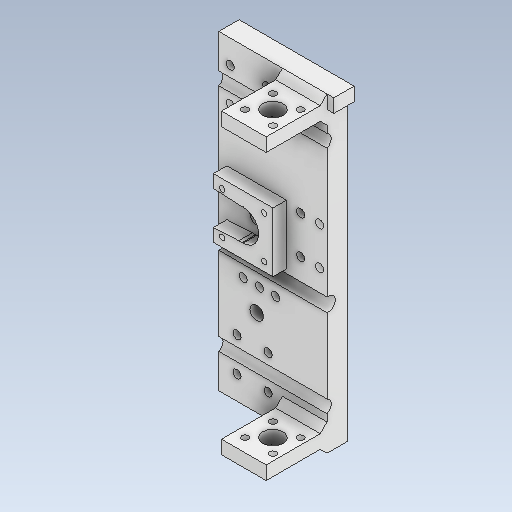
# Autodesk Inventor part: 0008-10-009 X Axis suport
Saved by Autodesk Inventor 2020 (Build 240168000, 168)
## iProperties
Created: 2021-02-27
Part Number: 0008-10-009 X Axis suport
Material: ABS Plastic
Document SubType Name: Modeling
Designer: Iulian Bors
Density: 1.06 g/cm^3
Appearance: Smooth - White
Mass: 294.815 g
Surface Area: 644.248 cm^2
Volume: 278.127 cm^3
Description: Supăort Axa X
Author: Iulian Bors
Subject: 009
Autodesk Inventor part; units mm, degrees
ref_plane "YZ Plane" through (0, 0, 0) normal (1, 0, 0) x (0, 1, 0)
ref_plane "XZ Plane" through (0, 0, 0) normal (0, 1, 0) x (-1, 0, 0)
ref_plane "XY Plane" through (0, 0, 0) normal (0, 0, 1) x (1, 0, 0)
sketch "Sketch1" plane through (0, 0, 0) normal (0, 0, 1) x (1, 0, 0)
  line L0 (-40, 115) -> (40, 115)
  line L1 (40, 115) -> (40, -115)
  line L2 (40, -115) -> (-40, -115)
  line L3 (-40, -115) -> (-40, 115)
  point P0 (0, 0)
  point P1 (0, 115)
  point P2 (-40, 0)
  dimension "d0" = 230
  dimension "d1" = 80
  constraints: 8 end point, 2 midpoint, 2 parallel, 1 horizontal, 1 horizontal alignment, 1 perpendicular, 1 vertical alignment
  measures "d0" distance of L2.end L0.start
  measures "d1" distance of L1.end L2.end
extrude "Extrusion1" add sketch "Sketch1" along normal blind 15
sketch "Sketch2" plane through (40, -115, 0) normal (1, 0, 0) x (0, 0, -1)
  circle A0 centre (-17, 30) radius 5.15
  circle A1 centre (-17, 200) radius 5.15
  line L0 (-15, 0) -> (-15, 230) projected
  line L1 (0, 230) -> (-15, 230) projected
  line L2 (0, 0) -> (-15, 0) projected
  point P0 (0, 115)
  dimension "d4" = 10.3
  dimension "d5" = 2
  dimension "d6" = 30
  dimension "d7" = 2
  dimension "d8" = 30
  constraints: 2 centre point, 1 equal radius
  measures "d4" diameter of A1
  measures "d5" distance from line of L0 A1.centre
  measures "d6" distance from line of L1 A1.centre
  measures "d7" distance from line of A0.centre L0
  measures "d8" distance from line of A0.centre L2
extrude "Extrusion2" cut sketch "Sketch2" against normal through all
sketch "Sketch3" plane through (-40, -115, 0) normal (-1, 0, 0) x (0, 0, 1)
  circle A0 centre (14, 95) radius 5.15
  line L0 (15, 195.2542) -> (15, 34.7458) projected
  line L1 (0, 0) -> (15, 0) projected
  point P0 (0, 115)
  dimension "d11" = 1
  dimension "d12" = 10.3
  dimension "d13" = 95
  constraints: 1 centre point
  measures "d11" distance from line of L0 A0.centre
  measures "d12" diameter of A0
  measures "d13" distance from line of A0.centre L1
extrude "Extrusion3" cut sketch "Sketch3" against normal through all
sketch "Sketch5" plane through (0, 0, 0) normal (0, 0, -1) x (-1, 0, 0)
  line L0 (34, -12) -> (-10, -12)
  line L1 (-10, -12) -> (-10, 32)
  line L2 (-10, 32) -> (34, 32)
  line L3 (34, 32) -> (34, -12)
  line L4 (34, -12) -> (-10, 32) construction
  line L5 (-10, -12) -> (34, 32) construction
  line L6 (-40, -115) -> (-40, 115)
  line L7 (-40, 115) -> (40, 115) projected
  line L8 (40, -115) -> (-40, -115) projected
  line L9 (-40, -115) -> (-40, 115) projected
  point P0 (12, 10)
  point P1 (12, -12)
  point P2 (0, -115)
  dimension "d17" = 44
  dimension "d43" = 105
  dimension "d64" = 52
  constraints: 14 end point, 4 midpoint, 3 perpendicular, 2 parallel
  measures "d17" distance of L0.start L0.end
  measures "d43" distance from line of L7 point (12, 10)
  measures "d64" distance from line of L6 point (12, 10)
extrude "Extrusion4" cut sketch "Sketch5" against normal blind 10
sketch "Sketch6" plane through (0, 0, 10) normal (0, 0, -1) x (-1, 0, 0)
  circle A0 centre (12, 10) radius 12.5
  line L0 (-40, -115) -> (-40, 115) projected
  line L1 (-40, 115) -> (40, 115) projected
  line L2 (40, -115) -> (-40, -115) projected
  point P0 (0, -115)
  dimension "d20" = 25
  dimension "d45" = 105
  dimension "d65" = 52
  constraints: 1 centre point, 1 coincident, 1 midpoint
  measures "d20" diameter of A0
  measures "d45" distance from line of L1 point (12, 10)
  measures "d65" distance from line of L0 point (12, 10)
extrude "Extrusion5" cut sketch "Sketch6" against normal blind 3
sketch "Sketch7" plane through (-12, 10, 13) normal (0, 0, -1) x (-1, 0, 0)
  circle A0 centre (0, 0) radius 5
  line L0 (-52, -125) -> (-52, 105) projected
  line L1 (-52, 105) -> (28, 105) projected
  line L2 (28, -125) -> (-52, -125) projected
  point P0 (-12, -125)
  dimension "d23" = 10
  dimension "d49" = 105
  dimension "d66" = 52
  constraints: 1 centre point, 1 coincident, 1 midpoint
  measures "d23" diameter of A0
  measures "d49" distance from line of L1 point (0, 0)
  measures "d66" distance from line of L0 point (0, 0)
extrude "Extrusion6" cut sketch "Sketch7" against normal through all
sketch "Sketch8" plane through (0, 0, 15) normal (0, 0, 1) x (1, 0, 0)
  line L0 (3.5, 25.5) -> (-27.5, 25.5) construction
  line L1 (-27.5, 25.5) -> (-27.5, -5.5) construction
  line L2 (-27.5, -5.5) -> (3.5, -5.5) construction
  line L3 (3.5, -5.5) -> (3.5, 25.5) construction
  line L4 (3.5, 25.5) -> (-27.5, -5.5) construction
  line L5 (-27.5, 25.5) -> (3.5, -5.5) construction
  line L6 (40, -115) -> (40, 115) projected
  line L7 (40, 115) -> (-40, 115) projected
  line L8 (-40, -115) -> (40, -115) projected
  point P0 (-12, 10)
  point P1 (-12, 10)
  point P2 (0, -115)
  dimension "d26" = 31
  dimension "d47" = 105
  dimension "d67" = 52
  constraints: 12 end point, 5 coincident, 3 midpoint, 2 parallel, 2 perpendicular, 1 horizontal
  measures "d26" distance of L1.end L2.end
  measures "d47" distance from line of L7 point (-12, 10)
  measures "d67" distance from line of point (-12, 10) L6
hole "Hole1" at (3.5, -5.5, 15) at (-27.5, -5.5, 15) at (-27.5, 25.5, 15) at (3.5, 25.5, 15) direction (0, 0, -1) diameter 4 depth 8 tip angle 118
sketch "Sketch9" plane through (0, 0, 15) normal (0, 0, 1) x (1, 0, 0)
  circle A0 centre (-27.5, 25.5) radius 2 projected
  circle A1 centre (3.5, -5.5) radius 2 projected
  circle A2 centre (-27.5, -5.5) radius 2
  circle A3 centre (3.5, 25.5) radius 2 projected
  circle A4 centre (-12, 10) radius 5
  line L0 (40, -25.052) -> (-40, -25.052) projected
  line L1 (-40, -25.052) -> (-40, -80.2542) projected
  line L2 (-40, -80.2542) -> (40, -80.2542) projected
  line L3 (40, -80.2542) -> (40, -25.052) projected
  line L4 (40, 80.2542) -> (-40, 80.2542) projected
  line L5 (-40, 80.2542) -> (-40, -14.948) projected
  line L6 (-40, -14.948) -> (40, -14.948) projected
  line L7 (40, 115) -> (-40, 115) projected
  line L8 (10, -12) -> (-34, -12)
  line L9 (-34, -12) -> (-34, 32)
  line L10 (-34, 32) -> (10, 32)
  line L11 (10, 32) -> (10, -12)
  line L12 (10, -12) -> (-34, 32) construction
  line L13 (-34, -12) -> (10, 32) construction
  line L14 (40, -14.948) -> (40, 80.2542) projected
  line L15 (-40, -115) -> (40, -115)
  line L16 (-40, -14.948) -> (40, -14.948) projected
  point P0 (-12, 10)
  point P1 (-12, -12)
  point P2 (0, -115)
  point P3 (10, 10)
  dimension "d52" = 105
  dimension "d55" = 44
  dimension "d68" = 52
  dimension "d69" = 44
  constraints: 14 end point, 6 midpoint, 3 perpendicular, 2 centre point, 2 parallel, 1 coincident, 1 horizontal, 1 horizontal alignment
  measures "d52" distance from line of L7 A4.centre
  measures "d55" distance of L8.start L8.end
  measures "d68" distance from line of A4.centre L14
  measures "d69" distance of L10.end L8.start
extrude "Extrusion7" add sketch "Sketch9" along normal blind 10 contours L8 L9 L10 L11
sketch "Sketch10" plane through (0, 0, 25) normal (0, 0, 1) x (1, 0, 0)
  arc A0 (-12, -1.5) -> (-12, 21.5) centre (-12, 10) ccw
  line L0 (-34, -1.5) -> (-12, -1.5)
  line L1 (-12, 21.5) -> (-34, 21.5)
  line L2 (-40, 80.2542) -> (-40, -14.948) projected
  line L3 (40, 115) -> (-40, 115) projected
  line L4 (-34, 32) -> (-34, -12) projected
  line L5 (-40, -115) -> (40, -115) projected
  line L6 (40, -14.948) -> (40, 80.2542) projected
  point P0 (0, -115)
  dimension "d38" = 23
  dimension "d54" = 105
  dimension "d70" = 52
  constraints: 4 end point, 2 perpendicular, 2 point on circle, 2 point on line, 2 tangent, 1 centre point, 1 coincident, 1 midpoint
  measures "d38" diameter of A0
  measures "d54" distance from line of point (-12, 10) L3
  measures "d70" distance from line of L6 point (-12, 10)
extrude "Extrusion8" cut sketch "Sketch10" against normal blind 10
chamfer "Chamfer1" distance 1 distance2 20 1 edges at (-34, -1.5, 20) measured on face at (-34, -5, 21.6667)
chamfer "Chamfer2" distance 1 distance2 20 1 edges at (-34, 21.5, 20) measured on face at (-34, 28.5, 18.3333)
fillet "Fillet3" radius 50 2 edges at (-14, -1.5, 20) (-14, 21.5, 20)
sketch "Sketch11" plane through (0, 0, 15) normal (0, 0, 1) x (1, 0, 0)
  line L0 (10, -94) -> (10, -100) projected
  line L1 (40, -110) -> (7, -110)
  line L2 (7, -110) -> (7, -100)
  line L3 (7, -100) -> (40, -100)
  line L4 (40, -100) -> (40, -110)
  line L5 (-40, -115) -> (40, -115) projected
  line L6 (40, -115) -> (40, -89.7458) projected
  point P0 (0, 0)
  dimension "d71" = 10
  dimension "d72" = 5
  dimension "d73" = 33
  constraints: 8 end point, 2 parallel, 1 collinear, 1 horizontal, 1 perpendicular
  measures "d71" distance of L3.end L1.start
  measures "d72" distance between parallel lines of L1 L5
  measures "d73" distance of L1.start L1.end
extrude "Extrusion9" add sketch "Sketch11" along normal blind 45
sketch "Sketch13" plane through (7, -100, 15) normal (0, 1, 0) x (1, 0, 0)
  circle A0 centre (28.253, -35.253) radius 2.5
  circle A1 centre (7.747, -35.253) radius 2.5
  circle A2 centre (7.747, -14.747) radius 2.5
  circle A3 centre (18, -25) radius 7.5
  circle A4 centre (28.253, -14.747) radius 2.5
  line L0 (33, 0) -> (33, -45) projected
  line L1 (33, -45) -> (0, -45) projected
  point P0 (-7, 15)
  dimension "d81" = 4.747
  dimension "d82" = 9.747
  dimension "d83" = 5
  dimension "d84" = 20.5061
  dimension "d85" = 20.5061
  dimension "d88" = 15
  dimension "d89" = 20
  dimension "d90" = 15
  constraints: 5 centre point, 3 equal radius, 2 horizontal alignment, 2 vertical alignment
  measures "d81" distance from line of L0 A0.centre
  measures "d82" distance from line of A0.centre L1
  measures "d83" diameter of A0
  measures "d84" distance of A1.centre A0.centre
  measures "d85" distance of A2.centre A1.centre
  measures "d88" distance from line of L0 A3.centre
  measures "d89" distance from line of A3.centre L1
  measures "d90" diameter of A3
extrude "Extrusion10" cut sketch "Sketch13" against normal through all
sketch "Sketch14" plane through (7, -110, 60) normal (0, -1, 0) x (1, 0, 0)
  circle A0 centre (7.747, -30.253) radius 2.5 projected
  circle A1 centre (28.253, -30.253) radius 2.5 projected
  line L0 (33, -45) -> (33, 0) projected
  line L1 (0, 0) -> (33, 0) projected
  line L2 (0, -45) -> (0, 0) projected
  circle A2 centre (18, -20) radius 7.5 projected
  circle A3 centre (7.747, -9.747) radius 2.5 projected
  circle A4 centre (28.253, -9.747) radius 2.5 projected
  circle A5 centre (28.253, -30.253) radius 2.5 projected
  circle A6 centre (28.253, -30.253) radius 4.5
  circle A7 centre (7.747, -30.253) radius 4.5
  line L3 (33, -45) -> (0, -45) projected
  point P0 (-7, -60)
  point P1 (25.7659, -30)
  point P2 (30.7402, -30)
  dimension "d94" = 9
  constraints: 2 centre point, 2 coincident, 1 equal radius
  measures "d94" diameter of A6
extrude "Extrusion11" cut sketch "Sketch14" along normal blind 35 contours A0 | A1 | A6 | A7
mirror "Mirror3" about plane through (0, 0, 0) normal (0, 1, 0) of "Extrusion9", "Extrusion10", "Extrusion11"
chamfer "Chamfer4" distance 5 angle 45 4 edges at (23.5, -110, 15) (23.5, -100, 15) (23.5, 100, 15) (23.5, 110, 15)
sketch "Sketch16" plane through (-40, 115, 0) normal (0, 1, 0) x (1, 0, 0)
  line L0 (85, -15) -> (80, -15)
  line L1 (80, -15) -> (80, 0)
  line L2 (80, 0) -> (85, 0)
  line L3 (85, 0) -> (85, -15)
  line L4 (80, 0) -> (80, -15) projected
  line L5 (80, -15) -> (47, -15) projected
  line L6 (80, 0) -> (0, 0) projected
  point P0 (40, 0)
  dimension "d101" = 5
  constraints: 8 end point, 3 collinear, 2 parallel, 1 horizontal, 1 perpendicular
  measures "d101" distance between parallel lines of L1 L3
extrude "Extrusion12" add sketch "Sketch16" against normal blind 10
sketch "Sketch17" plane through (0, 0, 0) normal (0, 0, -1) x (-1, 0, 0)
  arc A0 (27.7969, -100) -> (25.2031, -100) centre (26.5, -97.575) ccw projected
  arc A1 (4.7969, -100) -> (2.2031, -100) centre (3.5, -97.575) ccw projected
  circle A2 centre (3.5, -72.425) radius 2.75 projected
  circle A3 centre (26.5, -72.425) radius 2.75 projected
  circle A4 centre (22, -33.593) radius 2.75 projected
  circle A5 centre (10, -33.593) radius 2.75 projected
  circle A6 centre (-2, -33.593) radius 2.75 projected
  circle A7 centre (4.5, 72.425) radius 2.75 projected
  circle A8 centre (31.5, 72.425) radius 2.75 projected
  circle A9 centre (31.5, 97.575) radius 2.75 projected
  circle A10 centre (4.5, 97.575) radius 2.75 projected
  circle A11 centre (-20.5, 1) radius 2.5 projected
  circle A12 centre (-34.5, 1) radius 2.5 projected
  line L0 (-15, 20) -> (-40, 20) projected
  circle A13 centre (-34.5, 29) radius 2.5 projected
  circle A14 centre (-20.5, 29) radius 2.5 projected
  point P0 (0, 0)
hole "Hole2" at (-3.5, -97.575, 0) at (-26.5, -97.575, 0) at (-26.5, -72.425, 0) at (-3.5, -72.425, 0) at (2, -33.593, 0) at (-10, -33.593, 0) at (-22, -33.593, 0) at (-31.5, 72.425, 0) at (-4.5, 72.425, 0) at (-4.5, 97.575, 0) at (-31.5, 97.575, 0) at (20.5, 1, 0) at (34.5, 1, 0) at (34.5, 29, 0) at (20.5, 29, 0) direction (0, 0, 1) diameter 6 end through all
sketch "Sketch18" plane through (0, 0, 15) normal (0, 0, 1) x (1, 0, 0)
  circle A0 centre (-12, -51.1746) radius 5
  circle A1 centre (-12, 10) radius 6.1 projected
  point P0 (0, 0)
  dimension "d111" = 10
  dimension "d112" = 61.1746
  constraints: 1 centre point, 1 vertical alignment
  measures "d111" diameter of A0
  measures "d112" distance of A1.centre A0.centre
extrude "Extrusion13" cut sketch "Sketch18" against normal through all contours A0
equation "\"d7\" = d5"
equation "\"d8\" = d6"
equation "\"d45\" = d43"
equation "\"d65\" = d64"
equation "\"d49\" = d43"
equation "\"d66\" = d64"
equation "\"d47\" = d43"
equation "\"d67\" = d64"
equation "\"d52\" = d43"
equation "\"d68\" = d64"
equation "\"d54\" = d43"
equation "\"d70\" = d64"
body "Solid1"
